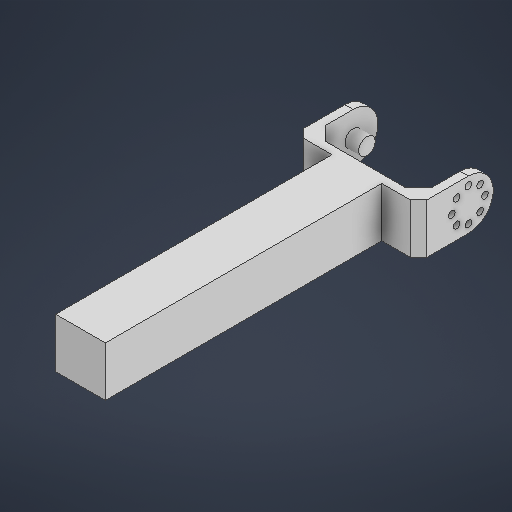
# Autodesk Inventor part: Arm2
Saved by Autodesk Inventor 2026 (Build 300175050, 175E)
## iProperties
Created: 2026-07-07
Part Number: Arm2
Material: 一般
Document SubType Name: Modeling
Designer: hanaj
Density: 1 g/cm^3
Appearance: 既定
Author: hanaj
Autodesk Inventor part; units mm, degrees
ref_plane "YZ Plane" through (0, 0, 0) normal (1, 0, 0) x (0, 1, 0)
ref_plane "XZ Plane" through (0, 0, 0) normal (0, 1, 0) x (-1, 0, 0)
ref_plane "XY Plane" through (0, 0, 0) normal (0, 0, 1) x (1, 0, 0)
sketch "スケッチ1" plane through (0, 0, 0) normal (1, 0, 0) x (0, 1, 0)
  circle A0 centre (0, 0) radius 9
  line L0 (9, 0) -> (-9, 0)
  line L1 (-9, 0) -> (-9, 18)
  line L2 (-9, 18) -> (9, 18)
  line L3 (9, 18) -> (9, 0)
  dimension "d0" = 18
  dimension "d1" = 18
  dimension "d2" = 18
  constraints: 8 end point, 2 parallel, 2 point on circle, 1 centre point, 1 coincident, 1 horizontal, 1 perpendicular
  measures "d0" diameter of A0
  measures "d1" distance of L0.end L1.end
  measures "d2" distance of L1.end L2.end
extrude "押し出し1" add sketch "スケッチ1" along normal blind 3
sketch "スケッチ2" plane through (3, 0, 0) normal (1, 0, 0) x (0, 0, -1)
  line L0 (-18, 9) -> (-18, -9) projected
  line L1 (-18, -9) -> (-15, -9)
  line L2 (-15, -9) -> (-15, 9)
  line L3 (-15, 9) -> (-18, 9)
  line L4 (-18, 9) -> (-18, -9)
  line L5 (0, 9) -> (-18, 9) projected
  point P0 (0, 0)
  dimension "d5" = 3
  constraints: 8 end point, 2 parallel, 1 collinear, 1 horizontal, 1 perpendicular
  measures "d5" distance between parallel lines of L2 L0
extrude "押し出し2" add sketch "スケッチ2" along normal blind 38.7
sketch "スケッチ3" plane through (41.7, 0, 0) normal (1, 0, 0) x (0, 0, -1)
  line L0 (-15, 9) -> (-15, -9) projected
  line L1 (-15, -9) -> (0, -9) projected
  arc A0 (0, -9) -> (0, 9) centre (0, 0) ccw projected
  line L2 (0, 9) -> (-15, 9) projected
  line L3 (-15, -9) -> (-15, 9) projected
  line L4 (-15, 9) -> (-18, 9) projected
  line L5 (-18, 9) -> (-18, -9) projected
  line L6 (-18, -9) -> (-15, -9) projected
extrude "押し出し3" add sketch "スケッチ3" along normal blind 3
sketch "スケッチ7" plane through (0, -9, 18) normal (0, 0, 1) x (1, 0, 0)
  line L0 (3, 0) -> (41.7, 0) projected
  line L1 (31.35, 18) -> (13.35, 18)
  line L2 (13.35, 18) -> (13.35, 0)
  line L3 (13.35, 0) -> (31.35, 0)
  line L4 (31.35, 0) -> (31.35, 18)
  line L5 (31.35, 18) -> (13.35, 0) construction
  line L6 (13.35, 18) -> (31.35, 0) construction
  line L7 (0, 18) -> (44.7, 18) projected
  line L8 (44.7, 18) -> (44.7, 0) projected
  point P0 (0, 9)
  point P1 (22.35, 9)
  point P2 (31.35, 0)
  dimension "d23" = 18
  dimension "d24" = 22.35
  constraints: 12 end point, 2 midpoint, 2 parallel, 1 collinear, 1 horizontal, 1 perpendicular, 1 point on line
  measures "d23" distance between parallel lines of L2 L4
  measures "d24" distance from line of point (22.35, 9) L8
extrude "押し出し7" add sketch "スケッチ7" along normal blind 100
sketch "スケッチ8" plane through (44.7, 0, 0) normal (1, 0, 0) x (0, 0, -1)
  circle A0 centre (0, 0) radius 6 construction
  line L0 (7.1439, 0) -> (-7.1439, 0) construction
  point P0 (-6, 0)
  point P1 (-4.2426, -4.2426)
  point P2 (0, -6)
  point P3 (4.2426, -4.2426)
  point P4 (6, 0)
  point P5 (4.2426, 4.2426)
  point P6 (0, 6)
  point P7 (-4.2426, 4.2426)
  dimension "d27" = 12
  dimension "d30" = 360
  constraints: 2 end point, 1 coincident, 1 horizontal, 1 horizontal alignment, 1 midpoint, 1 point on line, 11 other
hole "穴1" at (44.7, 0, 6) at (44.7, -4.2426, 4.2426) at (44.7, -6, 0) at (44.7, -4.2426, -4.2426) at (44.7, 0, -6) at (44.7, 4.2426, -4.2426) at (44.7, 6, 0) at (44.7, 4.2426, 4.2426) direction (-1, 0, 0) diameter 2.4 depth 6.3 clearance for "Countersunk Flat Head Screw ISO 2009/7046" size "M2" standard "ISO"
sketch "スケッチ9" plane through (3, 0, 0) normal (1, 0, 0) x (0, 0, -1)
  circle A0 centre (0, 0) radius 3
  dimension "d39" = 6
  constraints: 1 centre point, 1 coincident
  measures "d39" diameter of A0
extrude "押し出し8" add sketch "スケッチ9" along normal blind 5
chamfer "面取り1" distance 5 angle 45 2 edges at (3, 0, 15) (41.7, 0, 15)
chamfer "面取り2" distance 3 angle 45 2 edges at (0, 0, 18) (44.7, 0, 18)
